Autodesk Inventor part; units mm, degrees
(part 2 of 2)
  point P60 (0.3012, -58.3139)
  point P61 (2.0883, -60.3972)
  point P62 (-2.1274, -60.3972)
  point P63 (-3.3881, -68.5849)
  point P64 (0.8276, -68.5849)
  point P65 (4.2412, -46.4151)
  point P66 (0.0255, -46.4151)
  point P67 (2.9805, -54.6028)
  point P68 (-1.2352, -54.6028)
  point P69 (10.7588, -68.5849)
  point P70 (12.0195, -60.3972)
  point P71 (12.5459, -70.6683)
  point P72 (14.9745, -68.5849)
  point P73 (14.1158, -41.4346)
  point P74 (9.81, -69.3988)
  point P75 (1.5258, -69.3988)
  point P76 (9.1684, -73.5654)
  point P77 (11.5971, -71.4821)
  point P78 (0.8842, -73.5654)
  point P79 (-0.9029, -71.4821)
  point P80 (-1.601, -70.6683)
  point P81 (5.8316, -41.4346)
  point P82 (43.6787, -55.4167)
  point P83 (47.5, -57.5)
  point P84 (51.9629, -55.4167)
  point P85 (51.3213, -59.5833)
  point P86 (43.0371, -59.5833)
  point P87 (52.9117, -54.6028)
  point P88 (45.19, -45.6012)
  point P89 (54.1724, -46.4151)
  point P90 (58.3881, -46.4151)
  point P91 (57.1274, -54.6028)
  point P92 (53.4742, -45.6012)
  point P93 (56.601, -44.3317)
  point P94 (47.5, -57.5)
  point P95 (54.6988, -56.6861)
  point P96 (53.75, -57.5)
  point P97 (54.4481, -58.3139)
  point P98 (56.2352, -60.3972)
  point P99 (41.25, -57.5)
  point P100 (40.3012, -58.3139)
  point P101 (42.0883, -60.3972)
  point P102 (37.8726, -60.3972)
  point P103 (36.6119, -68.5849)
  point P104 (40.8276, -68.5849)
  point P105 (44.2412, -46.4151)
  point P106 (40.0255, -46.4151)
  point P107 (42.9805, -54.6028)
  point P108 (38.7648, -54.6028)
  point P109 (50.7588, -68.5849)
  point P110 (52.0195, -60.3972)
  point P111 (52.5459, -70.6683)
  point P112 (54.9745, -68.5849)
  point P113 (54.1158, -41.4346)
  point P114 (49.81, -69.3988)
  point P115 (41.5258, -69.3988)
  point P116 (49.1684, -73.5654)
  point P117 (51.5971, -71.4821)
  point P118 (40.8842, -73.5654)
  point P119 (39.0971, -71.4821)
  point P120 (38.399, -70.6683)
  point P121 (45.8316, -41.4346)
  point P122 (23.6787, -55.4167)
  point P123 (27.5, -57.5)
  point P124 (31.9629, -55.4167)
  point P125 (31.3213, -59.5833)
  point P126 (23.0371, -59.5833)
  point P127 (32.9117, -54.6028)
  point P128 (25.19, -45.6012)
  point P129 (34.1724, -46.4151)
  point P130 (38.3881, -46.4151)
  point P131 (37.1274, -54.6028)
  point P132 (33.4742, -45.6012)
  point P133 (36.601, -44.3317)
  point P134 (27.5, -57.5)
  point P135 (34.6988, -56.6861)
  point P136 (33.75, -57.5)
  point P137 (34.4481, -58.3139)
  point P138 (36.2352, -60.3972)
  point P139 (21.25, -57.5)
  point P140 (20.3012, -58.3139)
  point P141 (22.0883, -60.3972)
  point P142 (17.8726, -60.3972)
  point P143 (16.6119, -68.5849)
  point P144 (20.8276, -68.5849)
  point P145 (24.2412, -46.4151)
  point P146 (20.0255, -46.4151)
  point P147 (22.9805, -54.6028)
  point P148 (18.7648, -54.6028)
  point P149 (30.7588, -68.5849)
  point P150 (32.0195, -60.3972)
  point P151 (32.5459, -70.6683)
  point P152 (34.9745, -68.5849)
  point P153 (34.1158, -41.4346)
  point P154 (29.81, -69.3988)
  point P155 (21.5258, -69.3988)
  point P156 (29.1684, -73.5654)
  point P157 (31.5971, -71.4821)
  point P158 (20.8842, -73.5654)
  point P159 (19.0971, -71.4821)
  point P160 (18.399, -70.6683)
  point P161 (25.8316, -41.4346)
  point P162 (27.5, -57.5)
  point P163 (19.8269, -58.7208)
  point P164 (35.496, -43.0435)
  point P165 (29.9971, -69.6169)
  point P166 (21.3502, -69.5494)
  point P167 (27.5, -89.0815)
  dimension "d24" = 1.25
  dimension "d25" = 4.1667
  dimension "d26" = 4.1667
  dimension "d27" = 12.5
  dimension "d28" = 12.5
  dimension "d29" = 0.625
  dimension "d30" = 14.1469
  dimension "d31" = 14.1469
  dimension "d32" = 14.1469
  dimension "d33" = 20
  dimension "d34" = 20
  dimension "d36" = 22.5
  dimension "d37" = 8
  constraints: 364 end point, 337 point on line, 336 point on circle, 168 centre point, 24 tangent, 11 equal radius, 8 collinear, 8 midpoint, 5 parallel, 4 coincident, 4 horizontal, 2 vertical alignment, 1 perpendicular, 961 other
  measures "d24" distance between parallel lines of L18 L21
  measures "d25" distance between parallel lines of L17 L24
  measures "d26" distance between parallel lines of L13 L12
  measures "d27" distance of L22.start L22.end
  measures "d28" distance of L20.start L20.end
  measures "d29" radius of A22
  measures "d30" distance of L18.start L42.start
  measures "d31" distance of L18.start L6.start
  measures "d32" distance of L24.start L2.start
  measures "d33" distance of point (23.679, -55.417) point (3.679, -55.417)
  measures "d34" distance of point (23.679, -55.417) point (43.679, -55.417)
  measures "d36" distance of L182.start point (27.5, -57.5)
  measures "d37" angle of L3 L182
extrude "Extrusion4" cut sketch "Sketch3" against normal blind 0.5 contours L6 A1 L28 A34 L35 A28 L36 A35 L26 A18 L39 A33 | L7 A4 L16 A13 L14 A15 L19 A37 L42 A9 L8 A3 | L9 A6 L43 A41 L44 A26 L32 A25 L31 A11 L29 A5 | L11 A8 L27 A10 L12 A14 L25 A22 L18 A17 L13 A7 | A19 L21 A20 L23 A21 L24 A39 L45 A38 L41 A40 L17 | L30 A30 L38 A31 L37 A29 L34 A32 L33 A27 L40 A23 | L57 A47 L60 A78 L87 A79 L88 A80 L59 A50 L58 A49 | L64 A54 L67 A56 L72 A60 L66 A52 L63 A83 L62 A51 | L93 A99 L115 A101 L116 A104 L94 A90 L101 A97 L113 A95 | L106 A124 L136 A123 L135 A108 L123 A109 L124 A111 L97 A84 | A85 L98 A110 L125 A107 L96 A86 L99 A87 L114 A100 L95 | L102 A89 L105 A120 L132 A121 L133 A122 L104 A92 L103 A91 | L126 A114 L128 A115 L127 A113 L129 A119 L130 A117 L131 A112 | L188 S0 S1 S2 L189 S3 S4 S5 S6 L190 S7 S8 S9 S10 S11 S12 L191 | L192 L193 S13 S14 S15 L194 L195 L196 S16 S17 S18 S19 L197 | L198 S20 S21 S22 L199 S23 S24 S25 S26 L200 S27 S28 S29 S30 S31 S32 L201 | L202 L203 L204 L205 L206 L207 L208 L209 | L210 L211 L212 L213 L214 L215 L216 L217 | L221 L222 L223 L224 L225 L226 L227 L228 L229 L230 L231 L232 | L233 L234 L235 L236 L237 L238 L239 L240 L241 L242 | L243 L244 L245 L246 L247 L248 L249 L250 | L254 L255 L256 L257 | S33 S34 S35 S36 | L258 L259 L260 L261 S42 S43 S44 S45 L262
hole "Hole1" at (27.5, 39, 89.0815) direction (0, -1, 0) diameter 2.5 depth 6 counterbore diameter 5 counterbore depth 3.5
pattern_circular "Circular Pattern1" count 2 over 360 about axis through (27.5, 0, 100) along (0, 0, 1) of "Extrusion4", "Hole1"
equation "\"d4\" = d1"
equation "\"d5\" = d1"
equation "\"d52\" = d1"
equation "\"d51\" = d50"
equation "\"d24\" = 0.1 * d27"
equation "\"d25\" = 0.333333 * d27"
equation "\"d26\" = d25"
equation "\"d28\" = d27"
equation "\"d29\" = 0.05 * d27"
equation "\"d34\" = d33"
body "Solid1"
